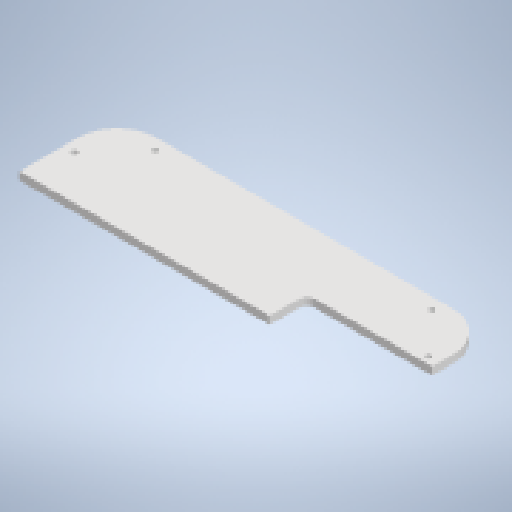
# Autodesk Inventor part: chest_cover_upper
Saved by Autodesk Inventor 2024.1 (Build 281209000, 209)
## iProperties
Created: 2024-02-29
Part Number: chest_cover_upper
Material: 一般
Document SubType Name: Modeling
Designer: hibik
Density: 1 g/cm^3
Appearance: 既定
Author: hibik
Autodesk Inventor part; units mm, degrees
ref_plane "YZ Plane" through (0, 0, 0) normal (1, 0, 0) x (0, 1, 0)
ref_plane "XZ Plane" through (0, 0, 0) normal (0, 1, 0) x (-1, 0, 0)
ref_plane "XY Plane" through (0, 0, 0) normal (0, 0, 1) x (1, 0, 0)
sketch "スケッチ1" plane through (0, 0, 0) normal (0, 1, 0) x (-1, 0, 0)
  line L0 (219.5254, 0) -> (0, 0)
  line L1 (0, 0) -> (0, -189.1417)
  line L2 (0, -189.1417) -> (219.5254, -189.1417)
  line L3 (219.5254, -189.1417) -> (219.5254, 0)
  constraints: 8 end point, 2 parallel, 1 coincident, 1 horizontal, 1 perpendicular
extrude "押し出し1" add sketch "スケッチ1" along normal blind 1.5
sketch "スケッチ2" plane through (0, 1.5, 0) normal (0, 1, 0) x (1, 0, 0)
  line L0 (-5.5, 10.4426) -> (-5.5, 0) projected
  line L1 (-5.5, 0) -> (0, 0) projected
  line L2 (0, 15) -> (0, 0) projected
  arc A0 (0, 15) -> (-10, 25) centre (-10, 15) ccw projected
  line L3 (-15, 25) -> (-10, 25) projected
  line L4 (-15, 25) -> (-15, 18) projected
  line L5 (-15, 18) -> (-5.5, 18) projected
  line L6 (-5.5, 18) -> (-5.5, 12.0415) projected
  arc A1 (-5.5, 10.4426) -> (-5.5, 12.0415) centre (-5.4702, 11.2421) ccw projected
  circle A2 centre (-12.6321, 22) radius 0.8 projected
  circle A3 centre (-83.3679, 22) radius 0.8 projected
  line L7 (-90.5, 0) -> (-90.5, 10.4426) projected
  arc A4 (-90.5, 12.0415) -> (-90.5, 10.4426) centre (-90.5298, 11.2421) ccw projected
  line L8 (-90.5, 12.0415) -> (-90.5, 18) projected
  line L9 (-90.5, 18) -> (-81, 18) projected
  line L10 (-81, 25) -> (-81, 18) projected
  line L11 (-81, 25) -> (-86, 25) projected
  arc A5 (-86, 25) -> (-96, 15) centre (-86, 15) ccw projected
  line L12 (-96, 15) -> (-96, 0) projected
  line L13 (-90.5, 0) -> (-96, 0) projected
  line L14 (-81, 25) -> (-15, 25)
  line L15 (-90.5, 0) -> (-5.5, 0)
  line L16 (-219.5254, 0) -> (0, 0) projected
  line L17 (0, 0) -> (0, 189.1417) projected
  line L18 (0, 189.1417) -> (-219.5254, 189.1417) projected
  line L19 (-219.5254, 189.1417) -> (-219.5254, 0) projected
  line L20 (-219.5254, 0) -> (0, 0) projected
  circle A6 centre (-93.25, 11.2421) radius 0.8
  circle A7 centre (-2.75, 11.2421) radius 0.8
  ellipse E0 centre (-7.5, 6.5336) end of major axis (-5.5, 6.5336) minor radius 1.9999 (-5.5, 6.5336) -> (-7.5, 8.5334) ccw projected
  line L21 (-7.5, 8.5334) -> (-29, 8.5334) projected
  ellipse E1 centre (-29, 6.5336) end of major axis (-27, 6.5336) minor radius 1.9999 (-29, 8.5334) -> (-31, 6.5336) ccw projected
  line L22 (-31, 6.5336) -> (-31, -8.9653) projected
  ellipse E2 centre (-29, -8.9653) end of major axis (-31, -8.9653) minor radius 1.9999 (-31, -8.9653) -> (-29, -10.9652) ccw projected
  line L23 (-29, -10.9652) -> (-1.5, -10.9652) projected
  line L24 (-1.5, -1.4659) -> (-1.5, -10.9652) projected
  line L25 (-5.5, -1.4659) -> (-1.5, -1.4659) projected
  line L26 (-5.5, -1.4659) -> (-5.5, 6.5336) projected
  line L27 (-9.5, -7.9654) -> (-28, -7.9654) projected
  line L28 (-28, -7.9654) -> (-28, 5.5336) projected
  line L29 (-28, 5.5336) -> (-9.5, 5.5336) projected
  line L30 (-9.5, 5.5336) -> (-9.5, -7.9654) projected
  line L31 (-32, 0) -> (0, 0)
  line L32 (0, 0) -> (0, 9.5334)
  line L33 (0, 9.5334) -> (-30, 9.5334)
  line L34 (-32, 7.5334) -> (-32, 0)
  arc A8 (-30, 9.5334) -> (-32, 7.5334) centre (-30, 7.5334) ccw
  point P0 (-2.75, 0)
  point P1 (-93.25, 0)
  dimension "d4" = 1.6
  dimension "d5" = 1.6
  dimension "d6" = 1
  dimension "d7" = 1
  dimension "d8" = 2
  constraints: 12 end point, 3 centre point, 2 horizontal, 2 horizontal alignment, 2 midpoint, 2 parallel, 2 point on circle, 2 point on line, 2 tangent, 2 vertical alignment, 1 collinear, 1 perpendicular, 3 other
  measures "d4" diameter of A6
  measures "d5" diameter of A7
  measures "d6" distance between parallel lines of L34 L22
  measures "d7" distance between parallel lines of L33 L21
  measures "d8" radius of A8
extrude "押し出し2" cut sketch "スケッチ2" against normal through all contours L0 L33 L2 L1 | E0 L21 E1 L22 L15 L34 A8 L33 L0 | L0 L15 L30 L29 L28 L22 E1 L21 E0 | L15 L28 L29 L30 | A0 L3 L14 L11 A5 L12 L16 L19 L18 L17 | A2 | A3 | A6 | A7
